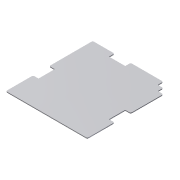
# Autodesk Inventor part: ProjectorPlate
Saved by Autodesk Inventor 2014 (Build 180170000, 170)
## iProperties
Created: 2014-08-10
Part Number: ProjectorPlate
Material: Generic
Document SubType Name: Modeling
Designer: Peele
Density: 1 g/cm^3
Appearance: White
Author: Peele
Autodesk Inventor part; units mm, degrees
ref_plane "YZ Plane" through (0, 0, 0) normal (1, 0, 0) x (0, 1, 0)
ref_plane "XZ Plane" through (0, 0, 0) normal (0, 1, 0) x (-1, 0, 0)
ref_plane "XY Plane" through (0, 0, 0) normal (0, 0, 1) x (1, 0, 0)
sketch "Sketch1" plane through (0, 0, 0) normal (0, 0, 1) x (1, 0, 0)
  line L0 (-187.5, -200) -> (187.5, -200)
  line L1 (187.5, -200) -> (187.5, 200)
  line L2 (187.5, 200) -> (-187.5, 200)
  line L3 (-187.5, 200) -> (-187.5, -200)
  line L4 (-187.5, -200) -> (187.5, 200) construction
  line L5 (187.5, -200) -> (-187.5, 200) construction
  point P0 (0, 0)
  dimension "d0" = 375
  dimension "d1" = 400
  constraints: 12 end point, 2 midpoint, 2 parallel, 1 horizontal, 1 perpendicular
  measures "d0" distance of L0.start L0.end
  measures "d1" distance of L0.end L1.end
extrude "Extrusion1" add sketch "Sketch1" along normal blind 4
sketch "Sketch6" plane through (0, 0, 0) normal (0, 0, -1) x (-1, 0, 0)
  line L0 (-187.5, 200) -> (-162.5, 200)
  line L1 (-162.5, 200) -> (-162.5, 175)
  line L2 (-162.5, 175) -> (-187.5, 175)
  line L3 (-187.5, 175) -> (-187.5, 200)
  line L4 (187.5, 200) -> (187.5, -200) projected
  line L5 (-187.5, 200) -> (187.5, 200) projected
  line L6 (-187.5, -200) -> (-187.5, 200) projected
  line L7 (-187.5, -25) -> (-162.5, -25)
  line L8 (-162.5, -25) -> (-162.5, -50)
  line L9 (-162.5, -50) -> (-187.5, -50)
  line L10 (-187.5, -50) -> (-187.5, -25)
  line L11 (187.5, -25) -> (162.5, -25)
  line L12 (162.5, -25) -> (162.5, -50)
  line L13 (162.5, -50) -> (187.5, -50)
  line L14 (187.5, -50) -> (187.5, -25)
  line L15 (62.5, 200) -> (37.5, 200)
  line L16 (37.5, 200) -> (37.5, 175)
  line L17 (37.5, 175) -> (62.5, 175)
  line L18 (62.5, 175) -> (62.5, 200)
  point P0 (0, 0)
  dimension "d22" = 25
  dimension "d25" = 200
  dimension "d26" = 200
  constraints: 32 end point, 8 parallel, 7 equal length, 4 horizontal, 4 perpendicular, 3 point on line, 1 collinear
  measures "d22" distance of L0.start L0.end
  measures "d25" distance between parallel lines of L2 L7
  measures "d26" distance between parallel lines of L1 L16
extrude "Extrusion6" cut sketch "Sketch6" against normal blind 4
sketch "Sketch7" plane through (0, 0, 0) normal (0, 0, -1) x (-1, 0, 0)
  line L0 (-162.5, -50) -> (-187.5, -50) projected
  line L1 (-187.5, -200) -> (-187.5, -50) projected
  line L2 (187.5, -50) -> (187.5, -200) projected
  line L3 (187.5, -50) -> (162.5, -50) projected
  line L4 (62.5, 200) -> (187.5, 200) projected
  line L5 (37.5, 175) -> (37.5, 200) projected
  line L6 (-162.5, 200) -> (37.5, 200) projected
  line L7 (-162.5, 175) -> (-187.5, 175) projected
  line L8 (-187.5, -25) -> (-187.5, 175) projected
  line L9 (-162.5, 175) -> (-187.5, 175)
  line L10 (-187.5, 175) -> (-187.5, 150)
  line L11 (-187.5, 150) -> (-162.5, 150)
  line L12 (-162.5, 150) -> (-162.5, 175)
  line L13 (-162.5, 175) -> (-137.5, 175)
  line L14 (-137.5, 175) -> (-137.5, 200)
  line L15 (-137.5, 200) -> (-162.5, 200)
  line L16 (-162.5, 200) -> (-162.5, 175)
  line L17 (37.5, 175) -> (12.5, 175)
  line L18 (12.5, 175) -> (12.5, 200)
  line L19 (12.5, 200) -> (37.5, 200)
  line L20 (37.5, 200) -> (37.5, 175)
  line L21 (62.5, 175) -> (87.5, 175)
  line L22 (87.5, 175) -> (87.5, 200)
  line L23 (87.5, 200) -> (62.5, 200)
  line L24 (62.5, 200) -> (62.5, 175)
  line L25 (187.5, -25) -> (162.5, -25)
  line L26 (162.5, -25) -> (162.5, 0)
  line L27 (162.5, 0) -> (187.5, 0)
  line L28 (187.5, 0) -> (187.5, -25)
  line L29 (162.5, -50) -> (187.5, -50)
  line L30 (187.5, -50) -> (187.5, -75)
  line L31 (187.5, -75) -> (162.5, -75)
  line L32 (162.5, -75) -> (162.5, -50)
  line L33 (-162.5, -50) -> (-187.5, -50)
  line L34 (-187.5, -50) -> (-187.5, -75)
  line L35 (-187.5, -75) -> (-162.5, -75)
  line L36 (-162.5, -75) -> (-162.5, -50)
  line L37 (-162.5, -25) -> (-187.5, -25)
  line L38 (-187.5, -25) -> (-187.5, 0)
  line L39 (-187.5, 0) -> (-162.5, 0)
  line L40 (-162.5, 0) -> (-162.5, -25)
  point P0 (0, 0)
  constraints: 64 end point, 16 parallel, 9 equal length, 8 horizontal, 8 perpendicular, 7 point on line
extrude "Extrusion7" cut sketch "Sketch7" against normal blind 4
fillet "Fillet3" radius 6 12 edges at (187.5, -200, 2) (187.5, -75, 2) (187.5, 0, 2) (187.5, 150, 2) (162.5, 175, 2) (137.5, 200, 2) (-12.5, 200, 2) (-87.5, 200, 2) (-187.5, 200, 2) (-187.5, -75, 2) (-187.5, -200, 2) (-187.5, 0, 2)
body "Solid1"
